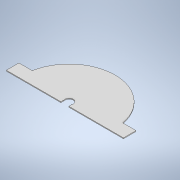
# Autodesk Inventor part: FlatRotationalTransfer
Saved by Autodesk Inventor 2020 (Build 240168000, 168)
## iProperties
Created: 2021-03-21
Part Number: FlatRotationalTransfer
Material: Generic
Document SubType Name: Sheet Metal
Designer: tdmp4
Density: 1 g/cm^3
Appearance: Default
Sheet Metal Rule: Default
Author: tdmp4
Autodesk Inventor part; units mm, degrees
ref_plane "YZ Plane" through (0, 0, 0) normal (1, 0, 0) x (0, 1, 0)
ref_plane "XZ Plane" through (0, 0, 0) normal (0, 1, 0) x (-1, 0, 0)
ref_plane "XY Plane" through (0, 0, 0) normal (0, 0, 1) x (1, 0, 0)
sketch "Sketch3" plane through (0, 0, 0) normal (0, 1, 0) x (-1, 0, 0)
  arc A0 (127.5964, -8.854) -> (151.8036, -8.854) centre (139.7, -12.7) ccw
  arc A1 (0, -12.7) -> (279.4, -12.7) centre (139.7, -12.7) ccw
  line L0 (279.4, -12.7) -> (279.4, 0)
  line L1 (279.4, 0) -> (151.8036, 0)
  line L2 (151.8036, 0) -> (151.8036, -8.854)
  line L3 (127.5964, 0) -> (0, 0)
  line L4 (0, 0) -> (0, -12.7)
  line L5 (127.5964, 0) -> (127.5964, -8.854)
  point P0 (0, -12.7)
  dimension "d9" = 279.4
  constraints: 12 end point, 4 point on circle, 3 vertical, 2 centre point, 2 perpendicular, 1 coincident, 1 point on line
  measures "d9" diameter of A1
extrude "Extrusion2" add sketch "Sketch3" along normal blind 2.54
sketch "Sketch6" plane through (-279.4, 0, -12.7) normal (-1, 0, 0) x (0, 0, 1)
  line L0 (12.7, 0) -> (3.846, 0) projected
  line L1 (0, 2.54) -> (-139.7, 2.54) projected
  line L2 (12.7, 0) -> (-25.4, 0)
  line L3 (-25.4, 0) -> (-25.4, 2.54)
  line L4 (-25.4, 2.54) -> (12.7, 2.54)
  line L5 (12.7, 2.54) -> (12.7, 0)
  dimension "d16" = 38.1
  constraints: 8 end point, 2 parallel, 1 horizontal, 1 perpendicular, 1 point on line
  measures "d16" distance of L3.end L4.end
extrude "Extrusion4" add sketch "Sketch6" along normal mid plane 76.2
sketch "Sketch7" plane through (0, 0, 0) normal (1, 0, 0) x (0, 0, -1)
  line L0 (38.1, 0) -> (0, 0) projected
  line L1 (0, 0) -> (38.1, 0)
  line L2 (38.1, 0) -> (38.1, 2.54)
  line L3 (38.1, 2.54) -> (0, 2.54)
  line L4 (0, 2.54) -> (0, 0)
  dimension "d19" = 38.1
  dimension "d20" = 2.54
  constraints: 8 end point, 2 parallel, 1 horizontal, 1 perpendicular
  measures "d19" distance of L3.end L2.end
  measures "d20" distance of L1.end L2.end
extrude "Extrusion5" add sketch "Sketch7" along normal mid plane 76.2
equation "\"BendRadius\" = Thickness"
equation "\"BendReliefWidth\" = Thickness"
equation "\"BendReliefDepth\" = 0.5 * Thickness"
equation "\"CornerReliefSize\" = 4 * Thickness"
equation "\"MinimumRemnant\" = 2 * Thickness"
equation "\"TransitionRadius\" = BendRadius"
equation "\"JacobiRadiusSize\" = Thickness"
equation "\"GapSize\" = Thickness"
equation "\"Thickness\" = 3.048"
body "Solid2"
